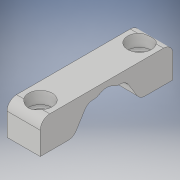
# Autodesk Inventor part: 3rd_phalanx_fingertip_holer
Saved by Autodesk Inventor 2017 (Build 210142000, 142)
## iProperties
Created: 2018-11-30
Part Number: 3rd_phalanx_fingertip_holer
Material: Generic
Document SubType Name: Modeling
Designer: tomas
Density: 1 g/cm^3
Appearance: Default
Author: tomas
## iProperties of the stored document 3rd_phalanx_fingertip_holer_3DPrint.ipt
Created: 2018-11-30
Part Number: 3rd_phalanx_fingertip_holer_3DPrint
Material: Generic
Document SubType Name: Modeling
Designer: tomas
Density: 1 g/cm^3
Appearance: Default
Author: tomas
Autodesk Inventor part; units mm, degrees
ref_plane "YZ Plane" through (0, 0, 0) normal (1, 0, 0) x (0, 1, 0)
ref_plane "XZ Plane" through (0, 0, 0) normal (0, 1, 0) x (-1, 0, 0)
ref_plane "XY Plane" through (0, 0, 0) normal (0, 0, 1) x (1, 0, 0)
sketch "Sketch1" plane through (0, 0, 0) normal (1, 0, 0) x (0, 1, 0)
  arc A0 (2.8, 0) -> (2.5667, 0.7739) centre (1.4, 0) ccw
  line L0 (0, 7.7385) -> (0, -8.1997) construction
  line L1 (-1.7375, 0) -> (6.7594, 0) construction
  line L2 (0, 3.5) -> (1.93, 2.2938)
  line L3 (2.4, 1.4458) -> (2.4, 1.3266)
  arc A1 (2.4, 1.4458) -> (1.93, 2.2938) centre (1.4, 1.4458) ccw
  line L4 (0, 3.5) -> (0, 7)
  line L5 (0, 7) -> (2.4, 7)
  line L6 (3.4, 6) -> (3.4, 0)
  arc A2 (3.4, 6) -> (2.4, 7) centre (2.4, 6) ccw
  arc A3 (2.4, 1.3266) -> (2.5667, 0.7739) centre (3.4, 1.3266) ccw
  arc A4 (2.5667, -0.7739) -> (2.8, 0) centre (1.4, 0) ccw
  line L7 (0, -3.5) -> (1.93, -2.2938)
  line L8 (2.4, -1.4458) -> (2.4, -1.3266)
  arc A5 (1.93, -2.2938) -> (2.4, -1.4458) centre (1.4, -1.4458) ccw
  line L9 (0, -3.5) -> (0, -7)
  line L10 (0, -7) -> (2.4, -7)
  line L11 (3.4, -6) -> (3.4, 0)
  arc A6 (2.4, -7) -> (3.4, -6) centre (2.4, -6) ccw
  arc A7 (2.5667, -0.7739) -> (2.4, -1.3266) centre (3.4, -1.3266) ccw
  point P0 (0, 0)
  point P1 (2.4, 2)
  point P2 (2.4, 0.9798)
  point P3 (3.4, 7)
  point P4 (0, -7.7385)
  dimension "d0" = 2.8
  dimension "d1" = 1
  dimension "d2" = 3.5
  dimension "d3" = 2
  dimension "d4" = 1
  dimension "d5" = 7
  dimension "d6" = 2
  dimension "d7" = 7
  dimension "d8" = 1
  dimension "d9" = 1
  constraints: 24 end point, 17 point on circle, 12 symmetric about line, 11 point on line, 8 centre point, 7 tangent, 3 vertical, 1 horizontal, 1 perpendicular, 4 other
  measures "d0" diameter of A0
  measures "d1" distance from line of L3 A0.centre
  measures "d2" distance of L2.start point (0, 0)
  measures "d3" distance from line of point (2.4, 2) L1
  measures "d4" radius of A1
  measures "d5" distance of L4.end point (0, 0)
  measures "d6" distance of L6.end A0.centre
  measures "d7" distance from line of point (3.4, 7) L1
  measures "d8" radius of A2
  measures "d9" radius of A3
extrude "Extrusion1" add sketch "Sketch1" along normal blind 3.5
sketch "Sketch2" plane through (0, 3.4, 6) normal (0, 1, 0) x (1, 0, 0)
  line L0 (0, 6) -> (3.5416, 6) construction
  line L1 (0, -1) -> (3.5, -1) projected
  line L2 (1.75, -1) -> (1.75, 12.2689) construction
  point P0 (1.75, 0.775)
  point P1 (1.75, 11.225)
  dimension "d12" = 5.225
  constraints: 4 end point, 1 horizontal, 1 midpoint, 1 point on line, 1 symmetric about line, 1 vertical
  measures "d12" distance from line of point (1.75, 0.775) L0
hole "Hole1" at (1.75, 3.4, 5.225) at (1.75, 3.4, -5.225) direction (0, -1, 0) diameter 1.5 end through all counterbore diameter 2.5 counterbore depth 1.3
fillet "Fillet1" radius 1 2 edges at (1.75, 0, 3.5) (1.75, 0, -3.5)
body "Solid1"
